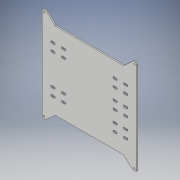
# Autodesk Inventor part: New Plate
Saved by Autodesk Inventor 2017 (Build 210142000, 142)
## iProperties
Created: 2017-03-05
Part Number: New Plate
Material: Generic
Document SubType Name: Modeling
Designer: gilef
Density: 1 g/cm^3
Appearance: Default
Author: gilef
Autodesk Inventor part; units mm, degrees
ref_plane "YZ Plane" through (0, 0, 0) normal (1, 0, 0) x (0, 1, 0)
ref_plane "XZ Plane" through (0, 0, 0) normal (0, 1, 0) x (-1, 0, 0)
ref_plane "XY Plane" through (0, 0, 0) normal (0, 0, 1) x (1, 0, 0)
sketch "Sketch1" plane through (0, 0, 0) normal (0, 0, 1) x (1, 0, 0)
  line L0 (0, 0) -> (218, 0)
  line L1 (218, 0) -> (218, 218)
  line L2 (218, 218) -> (0, 218)
  line L3 (0, 218) -> (0, 0)
  dimension "d0" = 218
  dimension "d1" = 218
  constraints: 8 end point, 2 parallel, 1 horizontal, 1 perpendicular
  measures "d0" distance of L1.end L2.end
  measures "d1" distance of L0.end L1.end
extrude "Extrusion1" add sketch "Sketch1" along normal blind 3
fillet "Fillet1" radius 3.175 4 edges at (218, 0, 1.5) (218, 218, 1.5) (0, 218, 1.5) (0, 0, 1.5)
sketch "Sketch2" plane through (0, 0, 3) normal (0, 0, 1) x (1, 0, 0)
  arc A0 (0, 3.175) -> (3.175, 0) centre (3.175, 3.175) ccw projected
  line L0 (3.175, 0) -> (214.825, 0) projected
  arc A1 (214.825, 0) -> (218, 3.175) centre (214.825, 3.175) ccw projected
  line L1 (218, 3.175) -> (218, 214.825) projected
  arc A2 (218, 214.825) -> (214.825, 218) centre (214.825, 214.825) ccw projected
  line L2 (214.825, 218) -> (3.175, 218) projected
  arc A3 (3.175, 218) -> (0, 214.825) centre (3.175, 214.825) ccw projected
  line L3 (0, 214.825) -> (0, 3.175) projected
  line L4 (214.825, 218) -> (3.175, 218) projected
  line L5 (30, 198) -> (188, 198)
  line L6 (3.175, 218) -> (8.175, 218)
  line L7 (8.175, 218) -> (30, 198)
  line L8 (214.825, 218) -> (209.825, 218)
  line L9 (188, 198) -> (209.825, 218)
  line L10 (0, 214.825) -> (0, 3.175) construction
  line L11 (0, 109) -> (218, 109) construction
  line L12 (30, 20) -> (188, 20)
  line L13 (3.175, 0) -> (8.175, 0)
  line L14 (8.175, 0) -> (30, 20)
  line L15 (214.825, 0) -> (209.825, 0)
  line L16 (188, 20) -> (209.825, 0)
  point P0 (0, 0)
  point P1 (5.675, 218)
  point P2 (212.325, 218)
  dimension "d5" = 20
  dimension "d6" = 30
  dimension "d7" = 30
  dimension "d8" = 20
  dimension "d9" = 5
  dimension "d10" = 5
  constraints: 22 end point, 4 midpoint, 4 symmetric about line, 2 horizontal alignment
  measures "d5" distance from line of L2 L5.start
  measures "d6" distance from line of L3 L5.start
  measures "d7" distance from line of L1 L5.end
  measures "d8" distance from line of L2 L5.end
  measures "d9" distance of L2.end L6.end
  measures "d10" distance of L2.start L8.end
extrude "Extrusion2" cut sketch "Sketch2" against normal through all contours L14 L12 L16 L0 | L2 L9 L5 L7
sketch "Sketch3" plane through (0, 0, 3) normal (0, 0, 1) x (1, 0, 0)
  line L0 (20.32, 162.4781) -> (30.1498, 162.4781) construction
  line L1 (22.5679, 160.2302) -> (27.9019, 160.2302)
  line L2 (27.9019, 164.726) -> (22.5679, 164.726)
  arc A0 (22.5679, 164.726) -> (22.5679, 160.2302) centre (22.5679, 162.4781) ccw
  arc A1 (27.9019, 160.2302) -> (27.9019, 164.726) centre (27.9019, 162.4781) ccw
  line L3 (0, 214.825) -> (0, 3.175) projected
  line L4 (3.175, 0) -> (8.175, 0) projected
  line L5 (209.825, 0) -> (214.825, 0) projected
  line L6 (218, 3.175) -> (218, 214.825) projected
  line L7 (214.825, 218) -> (209.825, 218) projected
  line L8 (8.175, 218) -> (3.175, 218) projected
  line L9 (8.175, 0) -> (30, 20) projected
  line L10 (30, 20) -> (188, 20) projected
  line L11 (188, 20) -> (209.825, 0) projected
  line L12 (209.825, 0) -> (214.825, 0) projected
  arc A2 (214.825, 0) -> (218, 3.175) centre (214.825, 3.175) ccw projected
  line L13 (218, 3.175) -> (218, 214.825) projected
  arc A3 (218, 214.825) -> (214.825, 218) centre (214.825, 214.825) ccw projected
  line L14 (214.825, 218) -> (209.825, 218) projected
  line L15 (209.825, 218) -> (188, 198) projected
  line L16 (188, 198) -> (30, 198) projected
  line L17 (30, 198) -> (8.175, 218) projected
  line L18 (8.175, 218) -> (3.175, 218) projected
  arc A4 (3.175, 218) -> (0, 214.825) centre (3.175, 214.825) ccw projected
  line L19 (0, 214.825) -> (0, 3.175) projected
  arc A5 (0, 3.175) -> (3.175, 0) centre (3.175, 3.175) ccw projected
  line L20 (3.175, 0) -> (8.175, 0) projected
  line L21 (20.32, 144.4822) -> (30.1498, 144.4822) construction
  line L22 (22.5679, 142.2343) -> (27.9019, 142.2343)
  line L23 (27.9019, 146.7301) -> (22.5679, 146.7301)
  arc A6 (22.5679, 146.7301) -> (22.5679, 142.2343) centre (22.5679, 144.4822) ccw
  arc A7 (27.9019, 142.2343) -> (27.9019, 146.7301) centre (27.9019, 144.4822) ccw
  line L24 (44.7548, 162.4781) -> (54.5846, 162.4781) construction
  line L25 (47.0027, 160.2302) -> (52.3367, 160.2302)
  line L26 (52.3367, 164.726) -> (47.0027, 164.726)
  arc A8 (47.0027, 164.726) -> (47.0027, 160.2302) centre (47.0027, 162.4781) ccw
  arc A9 (52.3367, 160.2302) -> (52.3367, 164.726) centre (52.3367, 162.4781) ccw
  line L27 (44.7548, 144.4822) -> (54.5846, 144.4822) construction
  line L28 (47.0027, 142.2343) -> (52.3367, 142.2343)
  line L29 (52.3367, 146.7301) -> (47.0027, 146.7301)
  arc A10 (47.0027, 146.7301) -> (47.0027, 142.2343) centre (47.0027, 144.4822) ccw
  arc A11 (52.3367, 142.2343) -> (52.3367, 146.7301) centre (52.3367, 144.4822) ccw
  line L30 (30, 198) -> (188, 198) construction
  line L31 (109, 198) -> (109, 20) construction
  line L32 (30, 20) -> (188, 20) construction
  line L33 (0, 214.825) -> (0, 3.175) construction
  line L34 (0, 109) -> (218, 109) construction
  line L35 (197.68, 162.4781) -> (187.8502, 162.4781) construction
  line L36 (195.4321, 160.2302) -> (190.0981, 160.2302)
  line L37 (190.0981, 164.726) -> (195.4321, 164.726)
  arc A12 (195.4321, 160.2302) -> (195.4321, 164.726) centre (195.4321, 162.4781) ccw
  arc A13 (190.0981, 164.726) -> (190.0981, 160.2302) centre (190.0981, 162.4781) ccw
  line L38 (197.68, 144.4822) -> (187.8502, 144.4822) construction
  line L39 (195.4321, 142.2343) -> (190.0981, 142.2343)
  line L40 (190.0981, 146.7301) -> (195.4321, 146.7301)
  arc A14 (195.4321, 142.2343) -> (195.4321, 146.7301) centre (195.4321, 144.4822) ccw
  arc A15 (190.0981, 146.7301) -> (190.0981, 142.2343) centre (190.0981, 144.4822) ccw
  line L41 (173.2452, 162.4781) -> (163.4154, 162.4781) construction
  line L42 (170.9973, 160.2302) -> (165.6633, 160.2302)
  line L43 (165.6633, 164.726) -> (170.9973, 164.726)
  arc A16 (170.9973, 160.2302) -> (170.9973, 164.726) centre (170.9973, 162.4781) ccw
  arc A17 (165.6633, 164.726) -> (165.6633, 160.2302) centre (165.6633, 162.4781) ccw
  line L44 (173.2452, 144.4822) -> (163.4154, 144.4822) construction
  line L45 (170.9973, 142.2343) -> (165.6633, 142.2343)
  line L46 (165.6633, 146.7301) -> (170.9973, 146.7301)
  arc A18 (170.9973, 142.2343) -> (170.9973, 146.7301) centre (170.9973, 144.4822) ccw
  arc A19 (165.6633, 146.7301) -> (165.6633, 142.2343) centre (165.6633, 144.4822) ccw
  line L47 (20.32, 55.5219) -> (30.1498, 55.5219) construction
  line L48 (22.5679, 57.7698) -> (27.9019, 57.7698)
  line L49 (27.9019, 53.274) -> (22.5679, 53.274)
  arc A20 (22.5679, 57.7698) -> (22.5679, 53.274) centre (22.5679, 55.5219) ccw
  arc A21 (27.9019, 53.274) -> (27.9019, 57.7698) centre (27.9019, 55.5219) ccw
  line L50 (20.32, 73.5178) -> (30.1498, 73.5178) construction
  line L51 (22.5679, 75.7657) -> (27.9019, 75.7657)
  line L52 (27.9019, 71.2699) -> (22.5679, 71.2699)
  arc A22 (22.5679, 75.7657) -> (22.5679, 71.2699) centre (22.5679, 73.5178) ccw
  arc A23 (27.9019, 71.2699) -> (27.9019, 75.7657) centre (27.9019, 73.5178) ccw
  line L53 (44.7548, 55.5219) -> (54.5846, 55.5219) construction
  line L54 (47.0027, 57.7698) -> (52.3367, 57.7698)
  line L55 (52.3367, 53.274) -> (47.0027, 53.274)
  arc A24 (47.0027, 57.7698) -> (47.0027, 53.274) centre (47.0027, 55.5219) ccw
  arc A25 (52.3367, 53.274) -> (52.3367, 57.7698) centre (52.3367, 55.5219) ccw
  line L56 (44.7548, 73.5178) -> (54.5846, 73.5178) construction
  line L57 (47.0027, 75.7657) -> (52.3367, 75.7657)
  line L58 (52.3367, 71.2699) -> (47.0027, 71.2699)
  arc A26 (47.0027, 75.7657) -> (47.0027, 71.2699) centre (47.0027, 73.5178) ccw
  arc A27 (52.3367, 71.2699) -> (52.3367, 75.7657) centre (52.3367, 73.5178) ccw
  line L59 (197.68, 55.5219) -> (187.8502, 55.5219) construction
  arc A28 (190.0981, 57.7698) -> (190.0981, 53.274) centre (190.0981, 55.5219) ccw
  line L60 (195.4321, 57.7698) -> (190.0981, 57.7698)
  arc A29 (195.4321, 53.274) -> (195.4321, 57.7698) centre (195.4321, 55.5219) ccw
  line L61 (190.0981, 53.274) -> (195.4321, 53.274)
  line L62 (170.9973, 75.7657) -> (165.6633, 75.7657)
  arc A30 (190.0981, 75.7657) -> (190.0981, 71.2699) centre (190.0981, 73.5178) ccw
  line L63 (190.0981, 71.2699) -> (195.4321, 71.2699)
  line L64 (195.4321, 75.7657) -> (190.0981, 75.7657)
  line L65 (197.68, 73.5178) -> (187.8502, 73.5178) construction
  arc A31 (195.4321, 71.2699) -> (195.4321, 75.7657) centre (195.4321, 73.5178) ccw
  arc A32 (165.6633, 75.7657) -> (165.6633, 71.2699) centre (165.6633, 73.5178) ccw
  line L66 (165.6633, 71.2699) -> (170.9973, 71.2699)
  line L67 (173.2452, 73.5178) -> (163.4154, 73.5178) construction
  line L68 (173.2452, 55.5219) -> (163.4154, 55.5219) construction
  arc A33 (170.9973, 53.274) -> (170.9973, 57.7698) centre (170.9973, 55.5219) ccw
  line L69 (165.6633, 53.274) -> (170.9973, 53.274)
  arc A34 (170.9973, 71.2699) -> (170.9973, 75.7657) centre (170.9973, 73.5178) ccw
  arc A35 (165.6633, 57.7698) -> (165.6633, 53.274) centre (165.6633, 55.5219) ccw
  line L70 (170.9973, 57.7698) -> (165.6633, 57.7698)
  line L71 (163.4154, 117.998) -> (173.2452, 117.998) construction
  line L72 (165.6633, 115.75) -> (170.9973, 115.75)
  line L73 (170.9973, 120.2459) -> (165.6633, 120.2459)
  arc A36 (165.6633, 120.2459) -> (165.6633, 115.75) centre (165.6633, 117.998) ccw
  arc A37 (170.9973, 115.75) -> (170.9973, 120.2459) centre (170.9973, 117.998) ccw
  line L74 (187.8502, 117.998) -> (197.68, 117.998) construction
  line L75 (190.0981, 115.75) -> (195.4321, 115.7501)
  line L76 (195.4321, 120.2458) -> (190.0981, 120.2459)
  arc A38 (190.0981, 120.2459) -> (190.0981, 115.75) centre (190.0981, 117.998) ccw
  arc A39 (195.4321, 115.7501) -> (195.4321, 120.2458) centre (195.4321, 117.998) ccw
  line L77 (163.4154, 100.0021) -> (173.2452, 100.0021) construction
  line L78 (165.6633, 97.7542) -> (170.9973, 97.7542)
  line L79 (170.9973, 102.2499) -> (165.6633, 102.2499)
  arc A40 (165.6633, 102.2499) -> (165.6633, 97.7542) centre (165.6633, 100.0021) ccw
  arc A41 (170.9973, 97.7542) -> (170.9973, 102.2499) centre (170.9973, 100.0021) ccw
  line L80 (187.8502, 100.0021) -> (197.68, 100.0021) construction
  line L81 (190.0981, 97.7542) -> (195.4321, 97.7542)
  line L82 (195.4321, 102.25) -> (190.0981, 102.2499)
  arc A42 (190.0981, 102.2499) -> (190.0981, 97.7542) centre (190.0981, 100.0021) ccw
  arc A43 (195.4321, 97.7542) -> (195.4321, 102.25) centre (195.4321, 100.0021) ccw
  point P0 (0, 0)
  point P1 (25.2349, 162.4781)
  point P2 (25.2349, 144.4822)
  point P3 (49.6697, 162.4781)
  point P4 (49.6697, 144.4822)
  point P5 (192.7651, 162.4781)
  point P6 (192.7651, 144.4822)
  point P7 (168.3303, 162.4781)
  point P8 (168.3303, 144.4822)
  point P9 (25.2349, 55.5219)
  point P10 (25.2349, 73.5178)
  point P11 (49.6697, 55.5219)
  point P12 (49.6697, 73.5178)
  point P13 (192.7651, 55.5219)
  point P14 (192.7651, 73.5178)
  point P15 (168.3303, 73.5178)
  point P16 (168.3303, 55.5219)
  point P17 (168.3303, 117.998)
  point P18 (192.7651, 117.998)
  point P19 (168.3303, 100.0021)
  point P20 (192.7651, 100.0021)
  dimension "d13" = 9.8298
  dimension "d14" = 4.4958
  dimension "d15" = 20.32
  dimension "d16" = 33.274
  dimension "d17" = 9.8298
  dimension "d18" = 4.4958
  dimension "d19" = 20.32
  dimension "d20" = 13.5001
  dimension "d21" = 33.274
  dimension "d22" = 4.4958
  dimension "d23" = 9.8298
  dimension "d24" = 14.605
  dimension "d25" = 13.5001
  dimension "d26" = 4.4958
  dimension "d27" = 9.8298
  dimension "d28" = 14.605
  dimension "d29" = 14.605
  dimension "d30" = 9.8298
  dimension "d31" = 9.8298
  dimension "d32" = 4.4958
  dimension "d33" = 4.4958
  dimension "d34" = 4.4958
  dimension "d35" = 4.4958
  dimension "d36" = 9.8298
  dimension "d37" = 9.8298
  dimension "d38" = 13.5001
  dimension "d39" = 20.32
  dimension "d40" = 21.9885
  dimension "d41" = 21.9885
  constraints: 164 end point, 128 point on circle, 108 symmetric about line, 44 point on line, 40 centre point, 32 tangent, 12 midpoint, 10 parallel, 4 horizontal, 4 vertical alignment, 24 other
  measures "d13" distance of L0.end L0.start
  measures "d14" distance between parallel lines of L1 L2
  measures "d15" distance from line of L3 L0.start
  measures "d16" distance between parallel lines of L16 L2
  measures "d17" distance of L21.end L21.start
  measures "d18" distance between parallel lines of L22 L23
  measures "d19" distance from line of L3 L21.start
  measures "d20" distance between parallel lines of L23 L1
  measures "d21" distance between parallel lines of L26 L16
  measures "d22" distance between parallel lines of L25 L26
  measures "d23" distance of L24.end L24.start
  measures "d24" distance of L0.end L24.start
  measures "d25" distance between parallel lines of L25 L29
  measures "d26" distance between parallel lines of L28 L29
  measures "d27" distance of L27.end L27.start
  measures "d28" distance of L21.end L27.start
  measures "d29" distance of L74.start L71.end
  measures "d30" distance of L71.end L71.start
  measures "d31" distance of L74.end L74.start
  measures "d32" distance between parallel lines of L78 L79
  measures "d33" distance between parallel lines of L72 L73
  measures "d34" distance between parallel lines of L75 L76
  measures "d35" distance between parallel lines of L81 L82
  measures "d36" distance of L80.end L80.start
  measures "d37" distance of L77.end L77.start
  measures "d38" distance between parallel lines of L79 L72
  measures "d39" distance from line of L13 L74.end
  measures "d40" distance between parallel lines of L73 L45
  measures "d41" distance between parallel lines of L62 L78
extrude "Extrusion3" cut sketch "Sketch3" against normal blind 25.4 contours A0 L2 A1 L1 | A6 L23 A7 L22 | A8 L26 A9 L25 | A10 L29 A11 L28 | L36 A13 L37 A12 | L39 A15 L40 A14 | L42 A17 L43 A16 | L45 A19 L46 A18 | L48 A21 L49 A20 | L51 A23 L52 A22 | L54 A25 L55 A24 | L57 A27 L58 A26 | L60 A29 L61 A28 | A34 L66 A32 L62 | L64 A31 L63 A30 | L69 A35 L70 A33 | A36 L73 A37 L72 | A38 L76 A39 L75 | A40 L79 A41 L78 | A42 L82 A43 L81
sketch "Sketch4" plane through (0, 0, 3) normal (0, 0, 1) x (1, 0, 0)
  circle A0 centre (5.0419, 5.1689) radius 1.7399
  line L0 (0, 214.825) -> (0, 3.175) projected
  line L1 (3.175, 0) -> (8.175, 0) projected
  circle A1 centre (212.9581, 5.1689) radius 1.7399
  line L2 (209.825, 0) -> (214.825, 0) projected
  line L3 (218, 3.175) -> (218, 214.825) projected
  circle A2 centre (212.9581, 212.8311) radius 1.7399
  line L4 (214.825, 218) -> (209.825, 218) projected
  circle A3 centre (5.0419, 212.8311) radius 1.7399
  line L5 (8.175, 218) -> (3.175, 218) projected
  point P0 (0, 0)
  dimension "d44" = 3.4798
  dimension "d45" = 3.302
  dimension "d46" = 3.429
  dimension "d47" = 3.4798
  dimension "d48" = 3.429
  dimension "d49" = 3.302
  dimension "d50" = 3.4798
  dimension "d51" = 3.429
  dimension "d52" = 3.302
  dimension "d53" = 3.4798
  dimension "d54" = 3.429
  dimension "d55" = 3.302
  constraints: 4 centre point
  measures "d44" diameter of A0
  measures "d45" distance edge to line of A0 L0
  measures "d46" distance edge to line of A0 L1
  measures "d47" diameter of A1
  measures "d48" distance edge to line of A1 L2
  measures "d49" distance edge to line of A1 L3
  measures "d50" diameter of A2
  measures "d51" distance edge to line of A2 L4
  measures "d52" distance edge to line of A2 L3
  measures "d53" diameter of A3
  measures "d54" distance edge to line of A3 L5
  measures "d55" distance edge to line of A3 L0
extrude "Extrusion4" cut sketch "Sketch4" against normal through all
equation "\"d17\" = d13"
equation "\"d18\" = d14"
equation "\"d19\" = d15"
equation "\"d21\" = d16"
equation "\"d22\" = d14"
equation "\"d23\" = d13"
equation "\"d25\" = d20"
equation "\"d26\" = d14"
equation "\"d27\" = d13"
equation "\"d28\" = d24"
equation "\"d29\" = d24"
equation "\"d30\" = d13"
equation "\"d31\" = d13"
equation "\"d32\" = d14"
equation "\"d33\" = d14"
equation "\"d34\" = d14"
equation "\"d35\" = d14"
equation "\"d38\" = d20"
equation "\"d39\" = d15"
equation "\"d40\" = d41"
body "Solid1"
